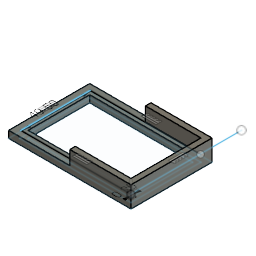
MORSE CASE (Autodesk Fusion 360 design; units mm, degrees)
part number: 2026-05-02-12-13-51-155
Autodesk Fusion 360 part; units mm, degrees
sketch "Sketch1" plane through (0, 0, 0) normal (0, 1, 0) x (1, 0, 0)
  line L0 (-29.5, 50) -> (50, 50)
  line L1 (50, 50) -> (50, 0)
  line L2 (50, 0) -> (-29.5, 0)
  line L3 (-29.5, 0) -> (-29.5, 50)
  line L4 (54, -4) -> (-33.5, -4)
  line L5 (-33.5, -4) -> (-33.5, 54)
  line L6 (-33.5, 54) -> (54, 54)
  line L7 (54, 54) -> (54, -4)
  line L8 (47, 3) -> (-26.5, 3)
  line L9 (-26.5, 3) -> (-26.5, 47)
  line L10 (-26.5, 47) -> (47, 47)
  line L11 (47, 47) -> (47, 3)
  dimension "d1" = 50
  dimension "d2" = 79.5
  dimension "d3" = -4
  dimension "d6" = 3
  constraint horizontal L0
  constraint vertical L1
  constraint horizontal L2
  constraint vertical L3
  measures "d1" distance of L0 L2
  measures "d2" distance of L1 L3
extrude "Extrude1" add sketch "Sketch1" along normal blind 5 contours L4 L5 L6 L7 makes body 1
extrude "Extrude2" add sketch "Sketch1" along normal blind 5 separate body contours L0 L1 L2 L3 makes body 2
sketch "Sketch2" plane through (0, 5, 0) normal (0, 1, 0) x (-1, 0, 0)
  line L0 (-50, 0) -> (29.5, 0)
  line L1 (29.5, 0) -> (29.5, -50)
  line L2 (29.5, -50) -> (-50, -50)
  line L3 (-50, -50) -> (-50, 0)
  line L4 (-54, -54) -> (33.5, -54)
  line L5 (33.5, -54) -> (33.5, 4)
  line L6 (33.5, 4) -> (-54, 4)
  line L7 (-54, 4) -> (-54, -54)
  line L8 (-10.25, -54) -> (-10.25, 4)
  constraint midpoint L4 L8.start
  constraint midpoint L6 L8.end
extrude "Extrude3" add sketch "Sketch2" along normal blind 10 contours L0 L2 L3 L4 L6 L7 L8 bodies 1 2
sketch "Sketch3" plane through (0, 5, 0) normal (0, 1, 0) x (-1, 0, 0)
  line L0 (-10.25, 4) -> (-10.25, 0)
  line L1 (-10.25, 0) -> (-50, 0)
  line L2 (-50, 0) -> (-50, -50)
  line L3 (-50, -50) -> (-10.25, -50)
  line L4 (-10.25, -50) -> (-10.25, -54)
  line L5 (-10.25, -54) -> (33.5, -54)
  line L6 (33.5, -54) -> (33.5, 4)
  line L7 (33.5, 4) -> (-10.25, 4)
  line L8 (26.5, -47) -> (-47, -47)
  line L9 (-47, -47) -> (-47, -3)
  line L10 (-47, -3) -> (26.5, -3)
  line L11 (26.5, -3) -> (26.5, -47)
  line L12 (-50, 0) -> (-50, -0.25)
  line L13 (-50, -0.25) -> (29, -0.25)
  line L14 (29, -0.25) -> (29, -49.75)
  line L15 (29, -49.75) -> (-50, -49.75)
  line L16 (-49.75, -79.25) -> (-49.75, -0.25)
  dimension "d11" = 0.25
  dimension "d12" = 49.5
  constraint coincident L1.end L2.start
  constraint perpendicular L1 L12
  constraint horizontal L13
  constraint vertical L14
  constraint horizontal L15
  constraint vertical L16
  measures "d11" distance of L1.end L12.end
  measures "d12" distance of L13 L15
